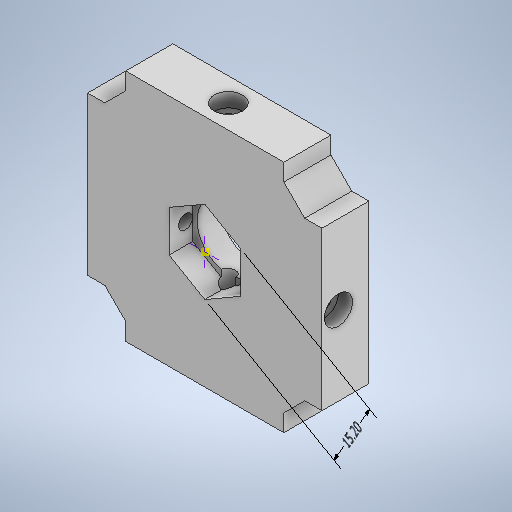
# Autodesk Inventor part: zhunzhiguan1
Saved by Autodesk Inventor 2025 (Build 290162000, 162)
## iProperties
Created: 2024-08-23
Part Number: zhunzhiguan1
Material: 常规
Document SubType Name: Sheet Metal
Designer: Leexi
Density: 1 g/cm^3
Sheet Metal Rule: 默认_mm
Appearance: 默认
Author: Leexi
Autodesk Inventor part; units mm, degrees
ref_plane "YZ Plane" through (0, 0, 0) normal (1, 0, 0) x (0, 1, 0)
ref_plane "XZ Plane" through (0, 0, 0) normal (0, 1, 0) x (-1, 0, 0)
ref_plane "XY Plane" through (0, 0, 0) normal (0, 0, 1) x (1, 0, 0)
sketch "草图1" plane through (0, 0, 0) normal (0, 0, 1) x (1, 0, 0)
  line L0 (24.9, 0) -> (24.9, 16.8)
  line L1 (24.9, 0) -> (41.7, 0) construction
  line L2 (24.9, 16.8) -> (21.24, 16.8)
  line L3 (21.24, 16.8) -> (16.7994, 21.2406)
  line L4 (16.7994, 21.2406) -> (16.7994, 24.9006)
  line L5 (16.7994, 24.9006) -> (-0.0006, 24.9006)
  line L6 (-0.0006, 24.9006) -> (-16.8006, 24.9006)
  line L7 (-16.8006, 24.9006) -> (-16.8006, 21.2406)
  line L8 (-16.8006, 21.2406) -> (-21.2413, 16.8)
  line L9 (-21.2413, 16.8) -> (-24.9013, 16.8)
  line L10 (-24.9013, 16.8) -> (-24.9013, 0)
  line L11 (-24.9013, 0) -> (-24.9013, -16.8)
  line L12 (-24.9013, -16.8) -> (-21.2413, -16.8)
  line L13 (-21.2413, -16.8) -> (-16.8006, -21.2406)
  line L14 (-16.8006, -21.2406) -> (-16.8006, -24.9006)
  line L15 (-16.8006, -24.9006) -> (16.7994, -24.9006)
  line L16 (16.7994, -24.9006) -> (16.7994, -21.2406)
  line L17 (16.7994, -21.2406) -> (21.24, -16.8)
  line L18 (21.24, -16.8) -> (24.9, -16.8)
  line L19 (24.9, -16.8) -> (24.9, 0)
  line L20 (-8.7757, 0) -> (-4.3879, 7.6)
  line L21 (-4.3879, 7.6) -> (4.3879, 7.6)
  line L22 (4.3879, 7.6) -> (8.7757, 0)
  line L23 (8.7757, 0) -> (4.3879, -7.6)
  line L24 (4.3879, -7.6) -> (-4.3879, -7.6)
  line L25 (-4.3879, -7.6) -> (-8.7757, 0)
  point P0 (0, 0)
  point P1 (0, 0)
  point P2 (0, 0)
  dimension "d61" = 15.2
  constraints: 52 end point, 10 perpendicular, 3 horizontal, 2 coincident, 2 collinear, 2 vertical, 1 parallel, 1 point on line, 13 other
  measures "d61" distance between parallel lines of L20 L23
extrude "拉伸1" add sketch "草图1" along normal blind 5 and the other way blind 5 contours L19 L18 L17 L16 L15 L14 L13 L12 L11 L10 L9 L8 L7 L6 L5 L4 L3 L2 L0 | L20 L21 L22 L23 L24 L25
sketch "草图2" plane through (0, 0, 5) normal (0, 0, 1) x (1, 0, 0)
  point P0 (0, 0)
sketch "草图3" plane through (0, 0, 5) normal (0, 0, 1) x (1, 0, 0)
  point P0 (0, 0)
sketch "草图4" plane through (0, 0, 5) normal (0, 0, 1) x (1, 0, 0)
  line L0 (7.6, -4.3879) -> (0, -8.7757)
  line L1 (0, -8.7757) -> (-7.6, -4.3879)
  line L2 (-7.6, -4.3879) -> (-7.6, 4.3879)
  line L3 (-7.6, 4.3879) -> (0, 8.7757)
  line L4 (0, 8.7757) -> (7.6, 4.3879)
  line L5 (7.6, 4.3879) -> (7.6, -4.3879)
  point P0 (0, 0)
  point P1 (0, 0)
  dimension "d30" = 15.2
  constraints: 12 end point, 1 coincident, 13 other
  measures "d30" distance between parallel lines of L2 L5
extrude "拉伸2" cut sketch "草图4" against normal blind 5
sketch "草图5" plane through (0, 0, 0) normal (0, 0, 1) x (1, 0, 0)
  point P0 (0, 0)
  point P1 (0, 0)
  constraints: 1 coincident
hole "孔1" at (0, 0, 0) direction (0, 0, -1) diameter 13.3 end through all
sketch "草图6" plane through (-24.9013, -16.8, 5) normal (-1, 0, 0) x (0, 0, 1)
  point P0 (-5, 16.8)
  point P1 (-3.5, 16.8)
hole "孔2" at (-24.9013, 0, 1.5) direction (1, 0, 0) diameter 2.98 end through all counterbore diameter 6 counterbore depth 3
sketch "草图7" plane through (24.9, -16.8, 5) normal (1, 0, 0) x (0, 0, -1)
  point P0 (5, 16.8)
  point P1 (3.5, 16.8)
hole "孔3" at (24.9, 0, 1.5) direction (-1, 0, 0) diameter 2.98 end through all counterbore diameter 6 counterbore depth 3
sketch "草图8" plane through (-16.8006, 24.9006, 5) normal (0, 1, 0) x (1, 0, 0)
  line L0 (24.4006, 5) -> (16.8006, 5) projected
  constraints: 1 coincident
hole "孔4" at (0, 24.9006, 0) direction (0, -1, 0) diameter 3 end through all counterbore diameter 6 counterbore depth 3
equation "\"d38\" = 厚度"
equation "\"折弯半径\" = 厚度"
equation "\"折弯释压宽度\" = 厚度"
equation "\"折弯释压深度\" = 0.5 * 厚度"
equation "\"拐角释压尺寸\" = 4 * 厚度"
equation "\"最小余量\" = 2 * 厚度"
equation "\"过渡半径\" = 折弯半径"
equation "\"Jacobi半径尺寸\" = 折弯半径"
equation "\"间隙大小\" = 厚度"
equation "\"厚度\" = 0.5"
